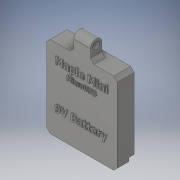
# Autodesk Inventor part: MMandBatteryCover
Saved by Autodesk Inventor 2018 (Build 220112000, 112)
## iProperties
Created: 2019-01-13
Part Number: MMandBatteryCover
Material: Generic
Document SubType Name: Modeling
Designer: tbrow
Density: 1 g/cm^3
Appearance: Default
Author: tbrow
Autodesk Inventor part; units mm, degrees
ref_plane "YZ Plane" through (0, 0, 0) normal (1, 0, 0) x (0, 1, 0)
ref_plane "XZ Plane" through (0, 0, 0) normal (0, 1, 0) x (-1, 0, 0)
ref_plane "XY Plane" through (0, 0, 0) normal (0, 0, 1) x (1, 0, 0)
sketch "Sketch1" plane through (0, 0, 0) normal (0, 0, 1) x (1, 0, 0)
  line L0 (0, 0) -> (0, 43.7642)
  line L1 (0, 43.7642) -> (14.478, 43.7642)
  line L2 (14.478, 43.7642) -> (14.478, 53.2892)
  line L3 (14.478, 53.2892) -> (23.368, 53.2892)
  line L4 (23.368, 53.2892) -> (23.368, 43.7642)
  line L5 (23.368, 43.7642) -> (37.846, 43.7642)
  line L6 (37.846, 43.7642) -> (37.846, 0)
  line L7 (37.846, 0) -> (0, 0)
  dimension "d0" = 8.89
  dimension "d1" = 9.525
  dimension "d2" = 14.478
  dimension "d3" = 14.478
  dimension "d4" = 43.7642
  constraints: 16 end point, 6 perpendicular, 2 point on line, 1 vertical
  measures "d0" distance of L2.end L3.end
  measures "d1" distance of L3.end L4.end
  measures "d2" distance of L0.end L1.end
  measures "d3" distance of L4.end L5.end
  measures "d4" distance of L0.start L0.end
extrude "Extrusion1" add sketch "Sketch1" along normal blind 6.2484
chamfer "Chamfer1" distance 1.905 angle 45 6 edges at (23.368, 43.7642, 3.1242) (14.478, 43.7642, 3.1242) (0, 43.7642, 3.1242) (37.846, 43.7642, 3.1242) (37.846, 0, 3.1242) (0, 0, 3.1242)
fillet "Fillet1" radius 3.1242 2 edges at (18.923, 53.2892, 6.2484) (18.923, 53.2892, 0)
sketch "Sketch2" plane through (23.368, 45.6692, 6.2484) normal (1, 0, 0) x (0, 0, -1)
  circle A0 centre (3.1242, 4.4958) radius 1.8542
  line L0 (0, 0) -> (0, 4.4958)
  line L1 (6.2484, 4.4958) -> (6.2484, 0)
  line L2 (0, 4.4958) -> (6.2484, 4.4958) construction
  line L3 (3.1242, 4.4958) -> (3.1242, 6.519489) construction
  point P0 (6.2484, -45.6692)
  dimension "d11" = 3.7084
  constraints: 4 end point, 1 centre point, 1 coincident, 1 horizontal, 1 midpoint, 1 vertical
  measures "d11" diameter of A0
extrude "Extrusion2" cut sketch "Sketch2" against normal through all
sketch "Sketch3" plane through (0, 0, 6.2484) normal (0, 0, 1) x (1, 0, 0)
  line L0 (4.569442, 38.044292) -> (33.276558, 38.044292) construction
  line L1 (33.276558, 38.044292) -> (33.276558, 28.917752) construction
  line L2 (33.276558, 28.917752) -> (4.569442, 28.917752) construction
  line L3 (4.569442, 28.917752) -> (4.569442, 38.044292) construction
  line L4 (23.368, 53.2892) -> (14.478, 53.2892)
  line L5 (18.923, 53.2892) -> (18.923, 0) construction
  line L6 (35.941, 0) -> (0, 0)
  line L7 (18.923, 38.044292) -> (18.923, 28.917752) construction
  line L8 (4.569442, 15.725753) -> (33.276558, 15.725753) construction
  line L9 (33.276558, 15.725753) -> (33.276558, 9.171238) construction
  line L10 (33.276558, 9.171238) -> (4.569442, 9.171238) construction
  line L11 (4.569442, 9.171238) -> (4.569442, 15.725753) construction
  line L12 (18.923, 15.725753) -> (18.923, 9.171238) construction
  line L13 (8.939503, 34.061391) -> (7.988547, 34.061391)
  line L14 (7.988547, 34.061391) -> (7.988547, 36.586982)
  line L15 (7.988547, 36.586982) -> (7.296942, 34.956772)
  line L16 (7.296942, 34.956772) -> (6.642388, 34.956772)
  line L17 (6.642388, 34.956772) -> (5.950783, 36.586982)
  line L18 (5.950783, 36.586982) -> (5.950783, 34.061391)
  line L19 (5.950783, 34.061391) -> (5.049227, 34.061391)
  line L20 (5.049227, 34.061391) -> (5.049227, 37.871391)
  line L21 (5.049227, 37.871391) -> (6.151472, 37.871391)
  line L22 (6.151472, 37.871391) -> (6.997453, 35.991091)
  line L23 (6.997453, 35.991091) -> (7.837258, 37.871391)
  line L24 (7.837258, 37.871391) -> (8.939503, 37.871391)
  line L25 (8.939503, 37.871391) -> (8.939503, 34.061391)
  spline S0 degree 2 poles (11.261318, 34.367055) (11.168693, 34.289867) (11.023579, 34.166366) (10.900078, 34.104616) knots 0 0 0 1 2 2 2
  spline S1 degree 2 poles (10.900078, 34.104616) (10.779665, 34.045953) (10.551189, 33.984203) (10.347412, 33.984203) knots 0 0 0 1 2 2 2
  spline S2 degree 2 poles (10.347412, 33.984203) (9.96456, 33.984203) (9.461294, 34.496731) (9.461294, 34.885759) knots 0 0 0 1 2 2 2
  spline S3 degree 2 poles (9.461294, 34.885759) (9.461294, 35.203773) (9.717558, 35.598976) (9.958385, 35.713214) knots 0 0 0 1 2 2 2
  spline S4 degree 2 poles (9.958385, 35.713214) (10.202299, 35.83054) (10.878466, 35.923166) (11.267493, 35.947866) knots 0 0 0 1 2 2 2
  line L26 (11.267493, 35.947866) -> (11.267493, 35.963303)
  spline S5 degree 2 poles (11.267493, 35.963303) (11.267493, 36.201042) (10.915516, 36.383206) (10.563539, 36.383206) knots 0 0 0 1 2 2 2
  spline S6 degree 2 poles (10.563539, 36.383206) (10.406075, 36.383206) (9.979997, 36.268968) (9.779309, 36.17943) knots 0 0 0 1 2 2 2
  line L27 (9.779309, 36.17943) -> (9.702121, 36.17943)
  line L28 (9.702121, 36.17943) -> (9.702121, 36.874122)
  spline S7 degree 2 poles (9.702121, 36.874122) (9.834884, 36.911172) (10.427688, 37.016148) (10.730265, 37.016148) knots 0 0 0 1 2 2 2
  spline S8 degree 2 poles (10.730265, 37.016148) (11.47127, 37.016148) (12.150524, 36.522145) (12.150524, 36.015791) knots 0 0 0 1 2 2 2
  line L29 (12.150524, 36.015791) -> (12.150524, 34.061391)
  line L30 (12.150524, 34.061391) -> (11.261318, 34.061391)
  line L31 (11.261318, 34.061391) -> (11.261318, 34.367055)
  line L32 (11.261318, 34.811658) -> (11.261318, 35.40755)
  spline S9 degree 2 poles (11.261318, 35.40755) (11.032842, 35.385937) (10.751877, 35.351974) (10.616027, 35.302574) knots 0 0 0 1 2 2 2
  spline S10 degree 2 poles (10.616027, 35.302574) (10.495613, 35.262436) (10.365937, 35.09571) (10.365937, 34.959859) knots 0 0 0 1 2 2 2
  spline S11 degree 2 poles (10.365937, 34.959859) (10.365937, 34.75917) (10.585151, 34.607882) (10.79819, 34.607882) knots 0 0 0 1 2 2 2
  spline S12 degree 2 poles (10.79819, 34.607882) (10.915516, 34.607882) (11.162518, 34.715945) (11.261318, 34.811658) knots 0 0 0 1 2 2 2
  spline S13 degree 2 poles (15.63016, 35.537226) (15.63016, 34.848708) (14.93238, 34.005815) (14.419852, 34.005815) knots 0 0 0 1 2 2 2
  spline S14 degree 2 poles (14.419852, 34.005815) (14.206813, 34.005815) (13.888798, 34.101529) (13.709722, 34.206504) knots 0 0 0 1 2 2 2
  line L33 (13.709722, 34.206504) -> (13.709722, 33.008546)
  line L34 (13.709722, 33.008546) -> (12.814341, 33.008546)
  line L35 (12.814341, 33.008546) -> (12.814341, 36.935872)
  line L36 (12.814341, 36.935872) -> (13.709722, 36.935872)
  line L37 (13.709722, 36.935872) -> (13.709722, 36.633295)
  spline S15 degree 2 poles (13.709722, 36.633295) (13.907323, 36.803109) (14.314876, 37.01306) (14.58349, 37.01306) knots 0 0 0 1 2 2 2
  spline S16 degree 2 poles (14.58349, 37.01306) (15.083669, 37.01306) (15.63016, 36.219568) (15.63016, 35.537226) knots 0 0 0 1 2 2 2
  spline S17 degree 2 poles (14.713166, 35.5187) (14.713166, 35.938603) (14.453814, 36.315281) (14.182113, 36.315281) knots 0 0 0 1 2 2 2
  spline S18 degree 2 poles (14.182113, 36.315281) (14.061699, 36.315281) (13.82396, 36.238093) (13.709722, 36.160905) knots 0 0 0 1 2 2 2
  line L38 (13.709722, 36.160905) -> (13.709722, 34.719033)
  spline S19 degree 2 poles (13.709722, 34.719033) (13.780735, 34.688157) (13.953636, 34.663457) (14.070962, 34.663457) knots 0 0 0 1 2 2 2
  spline S20 degree 2 poles (14.070962, 34.663457) (14.395151, 34.663457) (14.713166, 35.089535) (14.713166, 35.5187) knots 0 0 0 1 2 2 2
  line L39 (17.007194, 34.061391) -> (16.111813, 34.061391)
  line L40 (16.111813, 34.061391) -> (16.111813, 38.041205)
  line L41 (16.111813, 38.041205) -> (17.007194, 38.041205)
  line L42 (17.007194, 38.041205) -> (17.007194, 34.061391)
  spline S21 degree 2 poles (19.16537, 33.984203) (18.350265, 33.984203) (17.482672, 34.762258) (17.482672, 35.48165) knots 0 0 0 1 2 2 2
  spline S22 degree 2 poles (17.482672, 35.48165) (17.482672, 36.185605) (18.291602, 37.02541) (19.020257, 37.02541) knots 0 0 0 1 2 2 2
  spline S23 degree 2 poles (19.020257, 37.02541) (19.677899, 37.02541) (20.344803, 36.312193) (20.344803, 35.651464) knots 0 0 0 1 2 2 2
  line L43 (20.344803, 35.651464) -> (20.344803, 35.327274)
  line L44 (20.344803, 35.327274) -> (18.378053, 35.327274)
  spline S24 degree 2 poles (18.378053, 35.327274) (18.390403, 35.126585) (18.535516, 34.861059) (18.652842, 34.780783) knots 0 0 0 1 2 2 2
  spline S25 degree 2 poles (18.652842, 34.780783) (18.76708, 34.700508) (19.075832, 34.632582) (19.257996, 34.632582) knots 0 0 0 1 2 2 2
  spline S26 degree 2 poles (19.257996, 34.632582) (19.412372, 34.632582) (19.714949, 34.700508) (19.841537, 34.75917) knots 0 0 0 1 2 2 2
  spline S27 degree 2 poles (19.841537, 34.75917) (19.952688, 34.805483) (20.137939, 34.919721) (20.196602, 34.962947) knots 0 0 0 1 2 2 2
  line L45 (20.196602, 34.962947) -> (20.292315, 34.962947)
  line L46 (20.292315, 34.962947) -> (20.292315, 34.221942)
  spline S28 degree 2 poles (20.292315, 34.221942) (20.181165, 34.178717) (20.002088, 34.104616) (19.841537, 34.067566) knots 0 0 0 1 2 2 2
  spline S29 degree 2 poles (19.841537, 34.067566) (19.696424, 34.027428) (19.387672, 33.984203) (19.16537, 33.984203) knots 0 0 0 1 2 2 2
  spline S30 degree 2 poles (19.461772, 35.86759) (19.455597, 36.151642) (19.205508, 36.451132) (18.949244, 36.451132) knots 0 0 0 1 2 2 2
  spline S31 degree 2 poles (18.949244, 36.451132) (18.686805, 36.451132) (18.390403, 36.136204) (18.374965, 35.86759) knots 0 0 0 1 2 2 2
  line L47 (18.374965, 35.86759) -> (19.461772, 35.86759)
  line L48 (26.282105, 34.061391) -> (25.331149, 34.061391)
  line L49 (25.331149, 34.061391) -> (25.331149, 36.586982)
  line L50 (25.331149, 36.586982) -> (24.639544, 34.956772)
  line L51 (24.639544, 34.956772) -> (23.98499, 34.956772)
  line L52 (23.98499, 34.956772) -> (23.293385, 36.586982)
  line L53 (23.293385, 36.586982) -> (23.293385, 34.061391)
  line L54 (23.293385, 34.061391) -> (22.391829, 34.061391)
  line L55 (22.391829, 34.061391) -> (22.391829, 37.871391)
  line L56 (22.391829, 37.871391) -> (23.494074, 37.871391)
  line L57 (23.494074, 37.871391) -> (24.340055, 35.991091)
  line L58 (24.340055, 35.991091) -> (25.17986, 37.871391)
  line L59 (25.17986, 37.871391) -> (26.282105, 37.871391)
  line L60 (26.282105, 37.871391) -> (26.282105, 34.061391)
  line L61 (27.915403, 34.061391) -> (27.020022, 34.061391)
  line L62 (27.020022, 34.061391) -> (27.020022, 36.935872)
  line L63 (27.020022, 36.935872) -> (27.915403, 36.935872)
  line L64 (27.915403, 36.935872) -> (27.915403, 34.061391)
  line L65 (27.943191, 37.346512) -> (26.995322, 37.346512)
  line L66 (26.995322, 37.346512) -> (26.995322, 38.044292)
  line L67 (26.995322, 38.044292) -> (27.943191, 38.044292)
  line L68 (27.943191, 38.044292) -> (27.943191, 37.346512)
  line L69 (31.290063, 34.061391) -> (30.388507, 34.061391)
  line L70 (30.388507, 34.061391) -> (30.388507, 35.484738)
  spline S32 degree 2 poles (30.388507, 35.484738) (30.388507, 35.660726) (30.360719, 36.006529) (30.323669, 36.086804) knots 0 0 0 1 2 2 2
  spline S33 degree 2 poles (30.323669, 36.086804) (30.277356, 36.185605) (30.104455, 36.268968) (29.956254, 36.268968) knots 0 0 0 1 2 2 2
  spline S34 degree 2 poles (29.956254, 36.268968) (29.848191, 36.268968) (29.622802, 36.185605) (29.496214, 36.096067) knots 0 0 0 1 2 2 2
  line L71 (29.496214, 36.096067) -> (29.496214, 34.061391)
  line L72 (29.496214, 34.061391) -> (28.600833, 34.061391)
  line L73 (28.600833, 34.061391) -> (28.600833, 36.935872)
  line L74 (28.600833, 36.935872) -> (29.496214, 36.935872)
  line L75 (29.496214, 36.935872) -> (29.496214, 36.617858)
  spline S35 degree 2 poles (29.496214, 36.617858) (29.715427, 36.803109) (30.132243, 37.01306) (30.385419, 37.01306) knots 0 0 0 1 2 2 2
  spline S36 degree 2 poles (30.385419, 37.01306) (30.823847, 37.01306) (31.290063, 36.457307) (31.290063, 35.932428) knots 0 0 0 1 2 2 2
  line L76 (31.290063, 35.932428) -> (31.290063, 34.061391)
  line L77 (32.849261, 34.061391) -> (31.95388, 34.061391)
  line L78 (31.95388, 34.061391) -> (31.95388, 36.935872)
  line L79 (31.95388, 36.935872) -> (32.849261, 36.935872)
  line L80 (32.849261, 36.935872) -> (32.849261, 34.061391)
  line L81 (32.877048, 37.346512) -> (31.92918, 37.346512)
  line L82 (31.92918, 37.346512) -> (31.92918, 38.044292)
  line L83 (31.92918, 38.044292) -> (32.877048, 38.044292)
  line L84 (32.877048, 38.044292) -> (32.877048, 37.346512)
  line L85 (13.620853, 29.549355) -> (13.018581, 29.549355)
  line L86 (13.018581, 29.549355) -> (13.018581, 31.148896)
  line L87 (13.018581, 31.148896) -> (12.580565, 30.11643)
  line L88 (12.580565, 30.11643) -> (12.166014, 30.11643)
  line L89 (12.166014, 30.11643) -> (11.727997, 31.148896)
  line L90 (11.727997, 31.148896) -> (11.727997, 29.549355)
  line L91 (11.727997, 29.549355) -> (11.157012, 29.549355)
  line L92 (11.157012, 29.549355) -> (11.157012, 31.962355)
  line L93 (11.157012, 31.962355) -> (11.8551, 31.962355)
  line L94 (11.8551, 31.962355) -> (12.390888, 30.771498)
  line L95 (12.390888, 30.771498) -> (12.922765, 31.962355)
  line L96 (12.922765, 31.962355) -> (13.620853, 31.962355)
  line L97 (13.620853, 31.962355) -> (13.620853, 29.549355)
  line L98 (14.655275, 29.549355) -> (14.088201, 29.549355)
  line L99 (14.088201, 29.549355) -> (14.088201, 31.36986)
  line L100 (14.088201, 31.36986) -> (14.655275, 31.36986)
  line L101 (14.655275, 31.36986) -> (14.655275, 29.549355)
  line L102 (14.672874, 31.629932) -> (14.072557, 31.629932)
  line L103 (14.072557, 31.629932) -> (14.072557, 32.071859)
  line L104 (14.072557, 32.071859) -> (14.672874, 32.071859)
  line L105 (14.672874, 32.071859) -> (14.672874, 31.629932)
  spline S37 degree 2 poles (15.981057, 29.500469) (15.756182, 29.500469) (15.382695, 29.613884) (15.24386, 29.73121) knots 0 0 0 1 2 2 2
  spline S38 degree 2 poles (15.24386, 29.73121) (15.108935, 29.850491) (14.956412, 30.208335) (14.956412, 30.450808) knots 0 0 0 1 2 2 2
  spline S39 degree 2 poles (14.956412, 30.450808) (14.956412, 30.712836) (15.120668, 31.078501) (15.263414, 31.195827) knots 0 0 0 1 2 2 2
  spline S40 degree 2 poles (15.263414, 31.195827) (15.398339, 31.309242) (15.765959, 31.418746) (15.965413, 31.418746) knots 0 0 0 1 2 2 2
  spline S41 degree 2 poles (15.965413, 31.418746) (16.115981, 31.418746) (16.417117, 31.34835) (16.569641, 31.272088) knots 0 0 0 1 2 2 2
  line L106 (16.569641, 31.272088) -> (16.569641, 30.787142)
  line L107 (16.569641, 30.787142) -> (16.49729, 30.787142)
  spline S42 degree 2 poles (16.49729, 30.787142) (16.462092, 30.820384) (16.364321, 30.898601) (16.305658, 30.929888) knots 0 0 0 1 2 2 2
  spline S43 degree 2 poles (16.305658, 30.929888) (16.243084, 30.965086) (16.088605, 31.012016) (15.992789, 31.012016) knots 0 0 0 1 2 2 2
  spline S44 degree 2 poles (15.992789, 31.012016) (15.775737, 31.012016) (15.537174, 30.708925) (15.537174, 30.450808) knots 0 0 0 1 2 2 2
  spline S45 degree 2 poles (15.537174, 30.450808) (15.537174, 30.177048) (15.79138, 29.907199) (16.002566, 29.907199) knots 0 0 0 1 2 2 2
  spline S46 degree 2 poles (16.002566, 29.907199) (16.110115, 29.907199) (16.27046, 29.956084) (16.329123, 29.991282) knots 0 0 0 1 2 2 2
  spline S47 degree 2 poles (16.329123, 29.991282) (16.385831, 30.024524) (16.467959, 30.098831) (16.49729, 30.128162) knots 0 0 0 1 2 2 2
  line L108 (16.49729, 30.128162) -> (16.569641, 30.128162)
  line L109 (16.569641, 30.128162) -> (16.569641, 29.64126)
  spline S48 degree 2 poles (16.569641, 29.64126) (16.520755, 29.61975) (16.393652, 29.564998) (16.327168, 29.5474) knots 0 0 0 1 2 2 2
  spline S49 degree 2 poles (16.327168, 29.5474) (16.24504, 29.523934) (16.100338, 29.500469) (15.981057, 29.500469) knots 0 0 0 1 2 2 2
  line L110 (18.061634, 30.832117) -> (18.014703, 30.832117)
  spline S50 degree 2 poles (18.014703, 30.832117) (17.981461, 30.843849) (17.858269, 30.855582) (17.783963, 30.855582) knots 0 0 0 1 2 2 2
  spline S51 degree 2 poles (17.783963, 30.855582) (17.695968, 30.855582) (17.49847, 30.802785) (17.406565, 30.767588) knots 0 0 0 1 2 2 2
  line L111 (17.406565, 30.767588) -> (17.406565, 29.549355)
  line L112 (17.406565, 29.549355) -> (16.83949, 29.549355)
  line L113 (16.83949, 29.549355) -> (16.83949, 31.36986)
  line L114 (16.83949, 31.36986) -> (17.406565, 31.36986)
  line L115 (17.406565, 31.36986) -> (17.406565, 31.107832)
  spline S52 degree 2 poles (17.406565, 31.107832) (17.445673, 31.14303) (17.582553, 31.252534) (17.639261, 31.285776) knots 0 0 0 1 2 2 2
  spline S53 degree 2 poles (17.639261, 31.285776) (17.701835, 31.32293) (17.866091, 31.375726) (17.938442, 31.375726) knots 0 0 0 1 2 2 2
  spline S54 degree 2 poles (17.938442, 31.375726) (17.965818, 31.375726) (18.034258, 31.371815) (18.061634, 31.36986) knots 0 0 0 1 2 2 2
  line L116 (18.061634, 31.36986) -> (18.061634, 30.832117)
  spline S55 degree 2 poles (20.024885, 30.45863) (20.024885, 30.008881) (19.534072, 29.492647) (19.086279, 29.492647) knots 0 0 0 1 2 2 2
  spline S56 degree 2 poles (19.086279, 29.492647) (18.640441, 29.492647) (18.145717, 30.008881) (18.145717, 30.45863) knots 0 0 0 1 2 2 2
  spline S57 degree 2 poles (18.145717, 30.45863) (18.145717, 30.912289) (18.640441, 31.426567) (19.086279, 31.426567) knots 0 0 0 1 2 2 2
  spline S58 degree 2 poles (19.086279, 31.426567) (19.532117, 31.426567) (20.024885, 30.910334) (20.024885, 30.45863) knots 0 0 0 1 2 2 2
  spline S59 degree 2 poles (19.444122, 30.454719) (19.444122, 30.617019) (19.391326, 30.834072) (19.344395, 30.898601) knots 0 0 0 1 2 2 2
  spline S60 degree 2 poles (19.344395, 30.898601) (19.293554, 30.967041) (19.166451, 31.019838) (19.086279, 31.019838) knots 0 0 0 1 2 2 2
  spline S61 degree 2 poles (19.086279, 31.019838) (19.008062, 31.019838) (18.884869, 30.972908) (18.834028, 30.906423) knots 0 0 0 1 2 2 2
  spline S62 degree 2 poles (18.834028, 30.906423) (18.785143, 30.843849) (18.72648, 30.622886) (18.72648, 30.454719) knots 0 0 0 1 2 2 2
  spline S63 degree 2 poles (18.72648, 30.454719) (18.72648, 30.288507) (18.781232, 30.083187) (18.826207, 30.020613) knots 0 0 0 1 2 2 2
  spline S64 degree 2 poles (18.826207, 30.020613) (18.871181, 29.95804) (19.008062, 29.899377) (19.09019, 29.899377) knots 0 0 0 1 2 2 2
  spline S65 degree 2 poles (19.09019, 29.899377) (19.15863, 29.899377) (19.299421, 29.95804) (19.34244, 30.016703) knots 0 0 0 1 2 2 2
  spline S66 degree 2 poles (19.34244, 30.016703) (19.391326, 30.085143) (19.444122, 30.282641) (19.444122, 30.454719) knots 0 0 0 1 2 2 2
  spline S67 degree 2 poles (21.335023, 29.498514) (20.848121, 29.498514) (20.324066, 29.967817) (20.324066, 30.421477) knots 0 0 0 1 2 2 2
  line L117 (20.324066, 30.421477) -> (20.324066, 31.962355)
  line L118 (20.324066, 31.962355) -> (20.930249, 31.962355)
  line L119 (20.930249, 31.962355) -> (20.930249, 30.456674)
  spline S68 degree 2 poles (20.930249, 30.456674) (20.930249, 30.204424) (21.119925, 29.95804) (21.335023, 29.95804) knots 0 0 0 1 2 2 2
  spline S69 degree 2 poles (21.335023, 29.95804) (21.544254, 29.95804) (21.739797, 30.194647) (21.739797, 30.456674) knots 0 0 0 1 2 2 2
  line L120 (21.739797, 30.456674) -> (21.739797, 31.962355)
  line L121 (21.739797, 31.962355) -> (22.34598, 31.962355)
  line L122 (22.34598, 31.962355) -> (22.34598, 30.423432)
  spline S70 degree 2 poles (22.34598, 30.423432) (22.34598, 29.977594) (21.835613, 29.498514) (21.335023, 29.498514) knots 0 0 0 1 2 2 2
  spline S71 degree 2 poles (23.556391, 29.506335) (23.27872, 29.506335) (22.860258, 29.613884) (22.680358, 29.692101) knots 0 0 0 1 2 2 2
  line L123 (22.680358, 29.692101) -> (22.680358, 30.266998)
  line L124 (22.680358, 30.266998) -> (22.73511, 30.266998)
  spline S72 degree 2 poles (22.73511, 30.266998) (22.916965, 30.112519) (23.353026, 29.946307) (23.558346, 29.946307) knots 0 0 0 1 2 2 2
  spline S73 degree 2 poles (23.558346, 29.946307) (23.611143, 29.946307) (23.781265, 29.969772) (23.832106, 29.993237) knots 0 0 0 1 2 2 2
  spline S74 degree 2 poles (23.832106, 29.993237) (23.89468, 30.020613) (23.982674, 30.12034) (23.982674, 30.200513) knots 0 0 0 1 2 2 2
  spline S75 degree 2 poles (23.982674, 30.200513) (23.982674, 30.292418) (23.839928, 30.405833) (23.742156, 30.431254) knots 0 0 0 1 2 2 2
  spline S76 degree 2 poles (23.742156, 30.431254) (23.618964, 30.464496) (23.339338, 30.521203) (23.216146, 30.564223) knots 0 0 0 1 2 2 2
  spline S77 degree 2 poles (23.216146, 30.564223) (22.936519, 30.661994) (22.694046, 30.996373) (22.694046, 31.246668) knots 0 0 0 1 2 2 2
  spline S78 degree 2 poles (22.694046, 31.246668) (22.694046, 31.584957) (23.266987, 32.005374) (23.697182, 32.005374) knots 0 0 0 1 2 2 2
  spline S79 degree 2 poles (23.697182, 32.005374) (23.912279, 32.005374) (24.338562, 31.91738) (24.506729, 31.843074) knots 0 0 0 1 2 2 2
  line L125 (24.506729, 31.843074) -> (24.506729, 31.291643)
  line L126 (24.506729, 31.291643) -> (24.453933, 31.291643)
  spline S80 degree 2 poles (24.453933, 31.291643) (24.319008, 31.407013) (23.931833, 31.565403) (23.728468, 31.565403) knots 0 0 0 1 2 2 2
  spline S81 degree 2 poles (23.728468, 31.565403) (23.648296, 31.565403) (23.523148, 31.541938) (23.452753, 31.510651) knots 0 0 0 1 2 2 2
  spline S82 degree 2 poles (23.452753, 31.510651) (23.396045, 31.48523) (23.313917, 31.383548) (23.313917, 31.320974) knots 0 0 0 1 2 2 2
  spline S83 degree 2 poles (23.313917, 31.320974) (23.313917, 31.227113) (23.444931, 31.119565) (23.632652, 31.076545) knots 0 0 0 1 2 2 2
  spline S84 degree 2 poles (23.632652, 31.076545) (23.753889, 31.049169) (23.978763, 30.996373) (24.107822, 30.951398) knots 0 0 0 1 2 2 2
  spline S85 degree 2 poles (24.107822, 30.951398) (24.358117, 30.859493) (24.602545, 30.554446) (24.602545, 30.304151) knots 0 0 0 1 2 2 2
  spline S86 degree 2 poles (24.602545, 30.304151) (24.602545, 29.944352) (24.037426, 29.506335) (23.556391, 29.506335) knots 0 0 0 1 2 2 2
  spline S87 degree 2 poles (26.841512, 30.288507) (26.841512, 30.108608) (26.704632, 29.836803) (26.591217, 29.746853) knots 0 0 0 1 2 2 2
  spline S88 degree 2 poles (26.591217, 29.746853) (26.454337, 29.639305) (26.129736, 29.549355) (25.877485, 29.549355) knots 0 0 0 1 2 2 2
  line L127 (25.877485, 29.549355) -> (24.913459, 29.549355)
  line L128 (24.913459, 29.549355) -> (24.913459, 31.962355)
  line L129 (24.913459, 31.962355) -> (25.764071, 31.962355)
  spline S89 degree 2 poles (25.764071, 31.962355) (26.030009, 31.962355) (26.303769, 31.921291) (26.42305, 31.856762) knots 0 0 0 1 2 2 2
  spline S90 degree 2 poles (26.42305, 31.856762) (26.554064, 31.788322) (26.681167, 31.55367) (26.681167, 31.401147) knots 0 0 0 1 2 2 2
  spline S91 degree 2 poles (26.681167, 31.401147) (26.681167, 31.225158) (26.505178, 30.949442) (26.348744, 30.884913) knots 0 0 0 1 2 2 2
  line L130 (26.348744, 30.884913) -> (26.348744, 30.873181)
  spline S92 degree 2 poles (26.348744, 30.873181) (26.573618, 30.82625) (26.841512, 30.534891) (26.841512, 30.288507) knots 0 0 0 1 2 2 2
  spline S93 degree 2 poles (26.215775, 30.298284) (26.215775, 30.411699) (26.125825, 30.538802) (26.035875, 30.572045) knots 0 0 0 1 2 2 2
  spline S94 degree 2 poles (26.035875, 30.572045) (25.981123, 30.593554) (25.787536, 30.597465) (25.62719, 30.597465) knots 0 0 0 1 2 2 2
  line L131 (25.62719, 30.597465) -> (25.515731, 30.597465)
  line L132 (25.515731, 30.597465) -> (25.515731, 29.989327)
  line L133 (25.515731, 29.989327) -> (25.548973, 29.989327)
  spline S95 degree 2 poles (25.548973, 29.989327) (25.783625, 29.989327) (25.963524, 29.995193) (26.057385, 30.036257) knots 0 0 0 1 2 2 2
  spline S96 degree 2 poles (26.057385, 30.036257) (26.139513, 30.07341) (26.215775, 30.21029) (26.215775, 30.298284) knots 0 0 0 1 2 2 2
  spline S97 degree 2 poles (26.065207, 31.281865) (26.065207, 31.340528) (26.004588, 31.46372) (25.942015, 31.491096) knots 0 0 0 1 2 2 2
  spline S98 degree 2 poles (25.942015, 31.491096) (25.883352, 31.518472) (25.719096, 31.522383) (25.556795, 31.522383) knots 0 0 0 1 2 2 2
  line L134 (25.556795, 31.522383) -> (25.515731, 31.522383)
  line L135 (25.515731, 31.522383) -> (25.515731, 31.010061)
  line L136 (25.515731, 31.010061) -> (25.591993, 31.010061)
  spline S99 degree 2 poles (25.591993, 31.010061) (25.746472, 31.010061) (25.871619, 31.015927) (25.938104, 31.047214) knots 0 0 0 1 2 2 2
  spline S100 degree 2 poles (25.938104, 31.047214) (26.010455, 31.082412) (26.065207, 31.201693) (26.065207, 31.281865) knots 0 0 0 1 2 2 2
  spline S101 degree 2 poles (7.656962, 13.956604) (7.656962, 13.471863) (7.431573, 12.662933) (7.193834, 12.372706) knots 0 0 0 1 2 2 2
  spline S102 degree 2 poles (7.193834, 12.372706) (6.946833, 12.079392) (6.218178, 11.764465) (5.687124, 11.764465) knots 0 0 0 1 2 2 2
  spline S103 degree 2 poles (5.687124, 11.764465) (5.508048, 11.764465) (5.119021, 11.810777) (5.054183, 11.829302) knots 0 0 0 1 2 2 2
  line L137 (5.054183, 11.829302) -> (5.054183, 12.576482)
  line L138 (5.054183, 12.576482) -> (5.128283, 12.576482)
  spline S104 degree 2 poles (5.128283, 12.576482) (5.199296, 12.539432) (5.464823, 12.459157) (5.696387, 12.459157) knots 0 0 0 1 2 2 2
  spline S105 degree 2 poles (5.696387, 12.459157) (5.884726, 12.459157) (6.233616, 12.557957) (6.357116, 12.66602) knots 0 0 0 1 2 2 2
  spline S106 degree 2 poles (6.357116, 12.66602) (6.48988, 12.780259) (6.662781, 13.116798) (6.693656, 13.369975) knots 0 0 0 1 2 2 2
  spline S107 degree 2 poles (6.693656, 13.369975) (6.48988, 13.243387) (6.137902, 13.107536) (5.875463, 13.107536) knots 0 0 0 1 2 2 2
  spline S108 degree 2 poles (5.875463, 13.107536) (5.680949, 13.107536) (5.31971, 13.212512) (5.171509, 13.323662) knots 0 0 0 1 2 2 2
  spline S109 degree 2 poles (5.171509, 13.323662) (4.973907, 13.474951) (4.742343, 13.959691) (4.742343, 14.342544) knots 0 0 0 1 2 2 2
  spline S110 degree 2 poles (4.742343, 14.342544) (4.742343, 14.642033) (4.94612, 15.145299) (5.131371, 15.330551) knots 0 0 0 1 2 2 2
  spline S111 degree 2 poles (5.131371, 15.330551) (5.316622, 15.515802) (5.853851, 15.725753) (6.184215, 15.725753) knots 0 0 0 1 2 2 2
  spline S112 degree 2 poles (6.184215, 15.725753) (6.517667, 15.725753) (7.033283, 15.540502) (7.218535, 15.345988) knots 0 0 0 1 2 2 2
  spline S113 degree 2 poles (7.218535, 15.345988) (7.434661, 15.129862) (7.656962, 14.444432) (7.656962, 13.956604) knots 0 0 0 1 2 2 2
  spline S114 degree 2 poles (6.709094, 14.09863) (6.709094, 14.410469) (6.604118, 14.811847) (6.508405, 14.922998) knots 0 0 0 1 2 2 2
  spline S115 degree 2 poles (6.508405, 14.922998) (6.443567, 15.006361) (6.276841, 15.077374) (6.181128, 15.077374) knots 0 0 0 1 2 2 2
  spline S116 degree 2 poles (6.181128, 15.077374) (6.094677, 15.077374) (5.934126, 15.009448) (5.860026, 14.922998) knots 0 0 0 1 2 2 2
  spline S117 degree 2 poles (5.860026, 14.922998) (5.795188, 14.848897) (5.702562, 14.561758) (5.702562, 14.391944) knots 0 0 0 1 2 2 2
  spline S118 degree 2 poles (5.702562, 14.391944) (5.702562, 14.206693) (5.798275, 13.968954) (5.878551, 13.897941) knots 0 0 0 1 2 2 2
  spline S119 degree 2 poles (5.878551, 13.897941) (5.961914, 13.826928) (6.168778, 13.771353) (6.298454, 13.771353) knots 0 0 0 1 2 2 2
  spline S120 degree 2 poles (6.298454, 13.771353) (6.406517, 13.771353) (6.631906, 13.830016) (6.702919, 13.860891) knots 0 0 0 1 2 2 2
  spline S121 degree 2 poles (6.702919, 13.860891) (6.702919, 13.888679) (6.709094, 13.993654) (6.709094, 14.09863) knots 0 0 0 1 2 2 2
  line L139 (11.4824, 15.648565) -> (10.173292, 11.838565)
  line L140 (10.173292, 11.838565) -> (9.176022, 11.838565)
  line L141 (9.176022, 11.838565) -> (7.866914, 15.648565)
  line L142 (7.866914, 15.648565) -> (8.858008, 15.648565)
  line L143 (8.858008, 15.648565) -> (9.688551, 13.064311)
  line L144 (9.688551, 13.064311) -> (10.516006, 15.648565)
  line L145 (10.516006, 15.648565) -> (11.4824, 15.648565)
  spline S122 degree 2 poles (16.416258, 13.005648) (16.416258, 12.721596) (16.200131, 12.29243) (16.021055, 12.150405) knots 0 0 0 1 2 2 2
  spline S123 degree 2 poles (16.021055, 12.150405) (15.804929, 11.980591) (15.2924, 11.838565) (14.89411, 11.838565) knots 0 0 0 1 2 2 2
  line L146 (14.89411, 11.838565) -> (13.371963, 11.838565)
  line L147 (13.371963, 11.838565) -> (13.371963, 15.648565)
  line L148 (13.371963, 15.648565) -> (14.715034, 15.648565)
  spline S124 degree 2 poles (14.715034, 15.648565) (15.134937, 15.648565) (15.56719, 15.583727) (15.755528, 15.481839) knots 0 0 0 1 2 2 2
  spline S125 degree 2 poles (15.755528, 15.481839) (15.962392, 15.373776) (16.163081, 15.003273) (16.163081, 14.762447) knots 0 0 0 1 2 2 2
  spline S126 degree 2 poles (16.163081, 14.762447) (16.163081, 14.48457) (15.885204, 14.04923) (15.638203, 13.947341) knots 0 0 0 1 2 2 2
  line L149 (15.638203, 13.947341) -> (15.638203, 13.928816)
  spline S127 degree 2 poles (15.638203, 13.928816) (15.993267, 13.854716) (16.416258, 13.394675) (16.416258, 13.005648) knots 0 0 0 1 2 2 2
  spline S128 degree 2 poles (15.428251, 13.021085) (15.428251, 13.200161) (15.286225, 13.40085) (15.144199, 13.453338) knots 0 0 0 1 2 2 2
  spline S129 degree 2 poles (15.144199, 13.453338) (15.057749, 13.487301) (14.752084, 13.493476) (14.498908, 13.493476) knots 0 0 0 1 2 2 2
  line L150 (14.498908, 13.493476) -> (14.322919, 13.493476)
  line L151 (14.322919, 13.493476) -> (14.322919, 12.533257)
  line L152 (14.322919, 12.533257) -> (14.375407, 12.533257)
  spline S130 degree 2 poles (14.375407, 12.533257) (14.745909, 12.533257) (15.029961, 12.54252) (15.178162, 12.607358) knots 0 0 0 1 2 2 2
  spline S131 degree 2 poles (15.178162, 12.607358) (15.307838, 12.66602) (15.428251, 12.882147) (15.428251, 13.021085) knots 0 0 0 1 2 2 2
  spline S132 degree 2 poles (15.190512, 14.574108) (15.190512, 14.666734) (15.094799, 14.861247) (14.995998, 14.904473) knots 0 0 0 1 2 2 2
  spline S133 degree 2 poles (14.995998, 14.904473) (14.903373, 14.947698) (14.644021, 14.953873) (14.387757, 14.953873) knots 0 0 0 1 2 2 2
  line L153 (14.387757, 14.953873) -> (14.322919, 14.953873)
  line L154 (14.322919, 14.953873) -> (14.322919, 14.144943)
  line L155 (14.322919, 14.144943) -> (14.443332, 14.144943)
  spline S134 degree 2 poles (14.443332, 14.144943) (14.687246, 14.144943) (14.884848, 14.154205) (14.989823, 14.203606) knots 0 0 0 1 2 2 2
  spline S135 degree 2 poles (14.989823, 14.203606) (15.104062, 14.259181) (15.190512, 14.44752) (15.190512, 14.574108) knots 0 0 0 1 2 2 2
  spline S136 degree 2 poles (18.497246, 12.14423) (18.404621, 12.067042) (18.259507, 11.943541) (18.136007, 11.88179) knots 0 0 0 1 2 2 2
  spline S137 degree 2 poles (18.136007, 11.88179) (18.015593, 11.823127) (17.787117, 11.761377) (17.58334, 11.761377) knots 0 0 0 1 2 2 2
  spline S138 degree 2 poles (17.58334, 11.761377) (17.200488, 11.761377) (16.697222, 12.273905) (16.697222, 12.662933) knots 0 0 0 1 2 2 2
  spline S139 degree 2 poles (16.697222, 12.662933) (16.697222, 12.980948) (16.953486, 13.37615) (17.194313, 13.490388) knots 0 0 0 1 2 2 2
  spline S140 degree 2 poles (17.194313, 13.490388) (17.438227, 13.607714) (18.114394, 13.70034) (18.503421, 13.72504) knots 0 0 0 1 2 2 2
  line L156 (18.503421, 13.72504) -> (18.503421, 13.740478)
  spline S141 degree 2 poles (18.503421, 13.740478) (18.503421, 13.978217) (18.151444, 14.16038) (17.799467, 14.16038) knots 0 0 0 1 2 2 2
  spline S142 degree 2 poles (17.799467, 14.16038) (17.642003, 14.16038) (17.215926, 14.046142) (17.015237, 13.956604) knots 0 0 0 1 2 2 2
  line L157 (17.015237, 13.956604) -> (16.938049, 13.956604)
  line L158 (16.938049, 13.956604) -> (16.938049, 14.651296)
  spline S143 degree 2 poles (16.938049, 14.651296) (17.070812, 14.688346) (17.663616, 14.793322) (17.966193, 14.793322) knots 0 0 0 1 2 2 2
  spline S144 degree 2 poles (17.966193, 14.793322) (18.707198, 14.793322) (19.386452, 14.299319) (19.386452, 13.792965) knots 0 0 0 1 2 2 2
  line L159 (19.386452, 13.792965) -> (19.386452, 11.838565)
  line L160 (19.386452, 11.838565) -> (18.497246, 11.838565)
  line L161 (18.497246, 11.838565) -> (18.497246, 12.14423)
  line L162 (18.497246, 12.588832) -> (18.497246, 13.184724)
  spline S145 degree 2 poles (18.497246, 13.184724) (18.26877, 13.163111) (17.987806, 13.129149) (17.851955, 13.079748) knots 0 0 0 1 2 2 2
  spline S146 degree 2 poles (17.851955, 13.079748) (17.731541, 13.03961) (17.601866, 12.872884) (17.601866, 12.737033) knots 0 0 0 1 2 2 2
  spline S147 degree 2 poles (17.601866, 12.737033) (17.601866, 12.536345) (17.821079, 12.385056) (18.034118, 12.385056) knots 0 0 0 1 2 2 2
  spline S148 degree 2 poles (18.034118, 12.385056) (18.151444, 12.385056) (18.398446, 12.493119) (18.497246, 12.588832) knots 0 0 0 1 2 2 2
  spline S149 degree 2 poles (21.149426, 11.78299) (20.602935, 11.78299) (20.102757, 12.233768) (20.102757, 12.746296) knots 0 0 0 1 2 2 2
  line L163 (20.102757, 12.746296) -> (20.102757, 14.089367)
  line L164 (20.102757, 14.089367) -> (19.760042, 14.089367)
  line L165 (19.760042, 14.089367) -> (19.760042, 14.713046)
  line L166 (19.760042, 14.713046) -> (20.102757, 14.713046)
  line L167 (20.102757, 14.713046) -> (20.102757, 15.534327)
  line L168 (20.102757, 15.534327) -> (20.998138, 15.534327)
  line L169 (20.998138, 15.534327) -> (20.998138, 14.713046)
  line L170 (20.998138, 14.713046) -> (21.862644, 14.713046)
  line L171 (21.862644, 14.713046) -> (21.862644, 14.089367)
  line L172 (21.862644, 14.089367) -> (20.998138, 14.089367)
  line L173 (20.998138, 14.089367) -> (20.998138, 13.067398)
  spline S150 degree 2 poles (20.998138, 13.067398) (20.998138, 12.91611) (21.004313, 12.690721) (21.041363, 12.601183) knots 0 0 0 1 2 2 2
  spline S151 degree 2 poles (21.041363, 12.601183) (21.078413, 12.511644) (21.260577, 12.406669) (21.433478, 12.406669) knots 0 0 0 1 2 2 2
  spline S152 degree 2 poles (21.433478, 12.406669) (21.507579, 12.406669) (21.739143, 12.468419) (21.785456, 12.493119) knots 0 0 0 1 2 2 2
  line L174 (21.785456, 12.493119) -> (21.862644, 12.493119)
  line L175 (21.862644, 12.493119) -> (21.862644, 11.863265)
  spline S153 degree 2 poles (21.862644, 11.863265) (21.71753, 11.826215) (21.390253, 11.78299) (21.149426, 11.78299) knots 0 0 0 1 2 2 2
  spline S154 degree 2 poles (23.326128, 11.78299) (22.779637, 11.78299) (22.279459, 12.233768) (22.279459, 12.746296) knots 0 0 0 1 2 2 2
  line L176 (22.279459, 12.746296) -> (22.279459, 14.089367)
  line L177 (22.279459, 14.089367) -> (21.936744, 14.089367)
  line L178 (21.936744, 14.089367) -> (21.936744, 14.713046)
  line L179 (21.936744, 14.713046) -> (22.279459, 14.713046)
  line L180 (22.279459, 14.713046) -> (22.279459, 15.534327)
  line L181 (22.279459, 15.534327) -> (23.17484, 15.534327)
  line L182 (23.17484, 15.534327) -> (23.17484, 14.713046)
  line L183 (23.17484, 14.713046) -> (24.039345, 14.713046)
  line L184 (24.039345, 14.713046) -> (24.039345, 14.089367)
  line L185 (24.039345, 14.089367) -> (23.17484, 14.089367)
  line L186 (23.17484, 14.089367) -> (23.17484, 13.067398)
  spline S155 degree 2 poles (23.17484, 13.067398) (23.17484, 12.91611) (23.181015, 12.690721) (23.218065, 12.601183) knots 0 0 0 1 2 2 2
  spline S156 degree 2 poles (23.218065, 12.601183) (23.255115, 12.511644) (23.437279, 12.406669) (23.61018, 12.406669) knots 0 0 0 1 2 2 2
  spline S157 degree 2 poles (23.61018, 12.406669) (23.684281, 12.406669) (23.915845, 12.468419) (23.962157, 12.493119) knots 0 0 0 1 2 2 2
  line L187 (23.962157, 12.493119) -> (24.039345, 12.493119)
  line L188 (24.039345, 12.493119) -> (24.039345, 11.863265)
  spline S158 degree 2 poles (24.039345, 11.863265) (23.894232, 11.826215) (23.566955, 11.78299) (23.326128, 11.78299) knots 0 0 0 1 2 2 2
  spline S159 degree 2 poles (25.87642, 11.761377) (25.061315, 11.761377) (24.193722, 12.539432) (24.193722, 13.258824) knots 0 0 0 1 2 2 2
  spline S160 degree 2 poles (24.193722, 13.258824) (24.193722, 13.962779) (25.002652, 14.802585) (25.731307, 14.802585) knots 0 0 0 1 2 2 2
  spline S161 degree 2 poles (25.731307, 14.802585) (26.388948, 14.802585) (27.055853, 14.089367) (27.055853, 13.428638) knots 0 0 0 1 2 2 2
  line L189 (27.055853, 13.428638) -> (27.055853, 13.104448)
  line L190 (27.055853, 13.104448) -> (25.089102, 13.104448)
  spline S162 degree 2 poles (25.089102, 13.104448) (25.101452, 12.90376) (25.246566, 12.638233) (25.363892, 12.557957) knots 0 0 0 1 2 2 2
  spline S163 degree 2 poles (25.363892, 12.557957) (25.47813, 12.477682) (25.786882, 12.409756) (25.969046, 12.409756) knots 0 0 0 1 2 2 2
  spline S164 degree 2 poles (25.969046, 12.409756) (26.123422, 12.409756) (26.425999, 12.477682) (26.552587, 12.536345) knots 0 0 0 1 2 2 2
  spline S165 degree 2 poles (26.552587, 12.536345) (26.663738, 12.582657) (26.848989, 12.696896) (26.907652, 12.740121) knots 0 0 0 1 2 2 2
  line L191 (26.907652, 12.740121) -> (27.003365, 12.740121)
  line L192 (27.003365, 12.740121) -> (27.003365, 11.999116)
  spline S166 degree 2 poles (27.003365, 11.999116) (26.892214, 11.955891) (26.713138, 11.88179) (26.552587, 11.84474) knots 0 0 0 1 2 2 2
  spline S167 degree 2 poles (26.552587, 11.84474) (26.407474, 11.804602) (26.098722, 11.761377) (25.87642, 11.761377) knots 0 0 0 1 2 2 2
  spline S168 degree 2 poles (26.172822, 13.644764) (26.166647, 13.928816) (25.916558, 14.228306) (25.660294, 14.228306) knots 0 0 0 1 2 2 2
  spline S169 degree 2 poles (25.660294, 14.228306) (25.397854, 14.228306) (25.101452, 13.913379) (25.086015, 13.644764) knots 0 0 0 1 2 2 2
  line L193 (25.086015, 13.644764) -> (26.172822, 13.644764)
  line L194 (29.445594, 13.863978) -> (29.371493, 13.863978)
  spline S170 degree 2 poles (29.371493, 13.863978) (29.319005, 13.882503) (29.124492, 13.901029) (29.007166, 13.901029) knots 0 0 0 1 2 2 2
  spline S171 degree 2 poles (29.007166, 13.901029) (28.868227, 13.901029) (28.556388, 13.817666) (28.411274, 13.76209) knots 0 0 0 1 2 2 2
  line L195 (28.411274, 13.76209) -> (28.411274, 11.838565)
  line L196 (28.411274, 11.838565) -> (27.515893, 11.838565)
  line L197 (27.515893, 11.838565) -> (27.515893, 14.713046)
  line L198 (27.515893, 14.713046) -> (28.411274, 14.713046)
  line L199 (28.411274, 14.713046) -> (28.411274, 14.299319)
  spline S172 degree 2 poles (28.411274, 14.299319) (28.473025, 14.354894) (28.689151, 14.527795) (28.778689, 14.580283) knots 0 0 0 1 2 2 2
  spline S173 degree 2 poles (28.778689, 14.580283) (28.87749, 14.638946) (29.136842, 14.722309) (29.25108, 14.722309) knots 0 0 0 1 2 2 2
  spline S174 degree 2 poles (29.25108, 14.722309) (29.294305, 14.722309) (29.402368, 14.716134) (29.445594, 14.713046) knots 0 0 0 1 2 2 2
  line L200 (29.445594, 14.713046) -> (29.445594, 13.863978)
  line L201 (32.468276, 14.713046) -> (31.020229, 10.785721)
  line L202 (31.020229, 10.785721) -> (30.056923, 10.785721)
  line L203 (30.056923, 10.785721) -> (30.492263, 11.909578)
  line L204 (30.492263, 11.909578) -> (29.439419, 14.713046)
  line L205 (29.439419, 14.713046) -> (30.378025, 14.713046)
  line L206 (30.378025, 14.713046) -> (30.983179, 12.909935)
  line L207 (30.983179, 12.909935) -> (31.548195, 14.713046)
  line L208 (31.548195, 14.713046) -> (32.468276, 14.713046)
  point P0 (37.846, 0)
  constraints: 6 end point, 5 midpoint, 2 collinear, 1 point on line, 4 other
emboss "Emboss1" sketch "Sketch3" operation add depth 0.508 direction (0, 0, -1)
sketch "Sketch4" plane through (0, 0, 0) normal (0, 0, -1) x (-1, 0, 0)
  line L0 (-25.273, 43.7642) -> (-35.941, 43.7642)
  line L1 (-37.846, 41.8592) -> (-35.941, 43.7642)
  line L2 (-37.846, 41.8592) -> (-37.846, 1.905)
  line L3 (-35.941, 0) -> (-37.846, 1.905)
  line L4 (-35.941, 0) -> (-1.905, 0)
  line L5 (0, 1.905) -> (-1.905, 0)
  line L6 (0, 1.905) -> (0, 41.8592)
  line L7 (-1.905, 43.7642) -> (0, 41.8592)
  line L8 (-1.905, 43.7642) -> (-12.573, 43.7642)
  line L9 (-25.273, 43.7642) -> (-12.573, 43.7642)
  line L10 (-12.573, 42.4942) -> (-2.431051, 42.4942)
  line L11 (-2.431051, 42.4942) -> (-1.27, 41.333149)
  line L12 (-1.27, 41.333149) -> (-1.27, 2.431051)
  line L13 (-1.27, 2.431051) -> (-2.431051, 1.27)
  line L14 (-2.431051, 1.27) -> (-35.414949, 1.27)
  line L15 (-35.414949, 1.27) -> (-36.576, 2.431051)
  line L16 (-36.576, 2.431051) -> (-36.576, 41.333149)
  line L17 (-36.576, 41.333149) -> (-35.414949, 42.4942)
  line L18 (-35.414949, 42.4942) -> (-25.273, 42.4942)
  line L19 (-25.273, 42.4942) -> (-12.573, 42.4942)
  line L20 (-36.576, 3.175) -> (-1.27, 3.175)
  line L21 (-36.576, 3.81) -> (-37.846, 3.81)
  line L22 (-37.846, 1.905) -> (-37.846, 41.8592)
  line L23 (-1.27, 3.81) -> (0, 3.81)
  dimension "d16" = 1.27
  dimension "d17" = 3.175
  dimension "d18" = 0.635
  constraints: 28 end point, 6 point on line, 2 collinear, 2 perpendicular, 1 horizontal, 9 other
  measures "d16" distance between parallel lines of L0 L18
  measures "d17" distance between parallel lines of L4 L20
  measures "d18" distance between parallel lines of L20 L21
extrude "Extrusion3" add sketch "Sketch4" along normal blind 2.794 contours L9 L8 L7 L6 L23 L12 L11 L10 L19 L18 L17 L16 L21 L2 L1 L0
equation "\"d3\" = d2"
body "Solid1"
